Autodesk Fusion 360 part; units mm, degrees
note: some values were not read from the file. Chosen so that the rebuilt part matches the saved one: which face or edge a step refers to; how an offset face is resized; which pieces of a blend or face edit are solid. Set by a fixed rule: which sketch regions a step uses.
(part 2 of 2)
sketch "Sketch41" plane through (0, 0, 152) normal (0, 0, 1) x (-1, 0, 0)
  circle A0 centre (0, 0) radius 37.5
  circle A1 centre (-35, 35) radius 4.5178
  circle A2 centre (35, -35) radius 4.5178
  circle A3 centre (35, 35) radius 4.5178
  circle A4 centre (-35, -35) radius 4.5178
  line L0 (-250.7522, -75) -> (250.25, -75)
  line L1 (250.25, -75) -> (250.25, 75)
  line L2 (250.25, 75) -> (-250.7522, 75)
  line L3 (-250.7522, 75) -> (-250.7522, -75)
  line L4 (250.25, -75) -> (237.75, -75)
  line L5 (237.75, -75) -> (237.75, -50)
  line L6 (237.75, -50) -> (250.25, -50)
  line L7 (250.25, -50) -> (250.25, -75)
  line L8 (250.25, 75) -> (237.75, 75)
  line L9 (237.75, 75) -> (237.75, 50)
  line L10 (237.75, 50) -> (250.25, 50)
  line L11 (250.25, 50) -> (250.25, 75)
  line L12 (237.75, 50) -> (237.75, 0)
  line L13 (-250.7522, -75) -> (-238.2522, -75)
  line L14 (-238.2522, -75) -> (-238.2522, -50)
  line L15 (-238.2522, -50) -> (-250.7522, -50)
  line L16 (-250.7522, -50) -> (-250.7522, -75)
  line L17 (-250.7522, 75) -> (-238.2522, 75)
  line L18 (-238.2522, 75) -> (-238.2522, 50)
  line L19 (-238.2522, 50) -> (-250.7522, 50)
  line L20 (-250.7522, 50) -> (-250.7522, 75)
  line L21 (-238.2522, 50) -> (-238.2522, 0)
  dimension "d300" = 12.5
  dimension "d301" = 25
  dimension "d302" = 12.5
  dimension "d303" = 25
  dimension "d304" = 50
  dimension "d305" = 12.5
  dimension "d306" = 25
  dimension "d307" = 12.5
  dimension "d308" = 25
  dimension "d309" = 50
  constraint horizontal L4
  constraint vertical L5
  constraint horizontal L6
  constraint vertical L7
  constraint coincident L0.end L1.start
  constraint horizontal L8
  constraint vertical L9
  constraint horizontal L10
  constraint vertical L11
  constraint coincident L1.end L2.start
  constraint perpendicular L10 L12
  constraint horizontal L13
  constraint vertical L14
  constraint horizontal L15
  constraint vertical L16
  constraint coincident L0.start L3.end
  constraint horizontal L17
  constraint vertical L18
  constraint horizontal L19
  constraint vertical L20
  constraint coincident L2.end L3.start
  constraint perpendicular L19 L21
  measures "d300" distance of L0.end L4.end
  measures "d301" distance of L0.end L6.end
  measures "d302" distance of L1.end L8.end
  measures "d303" distance of L1.end L10.end
  measures "d304" distance of L9.end L12.end
  measures "d305" distance of L0.start L13.end
  measures "d306" distance of L0.start L15.end
  measures "d307" distance of L2.end L17.end
  measures "d308" distance of L2.end L19.end
  measures "d309" distance of L18.end L21.end
hole "Hole23" at (238.2522, 50, 152) at (238.2522, 0, 152) at (238.2522, -50, 152) at (-237.75, -50, 152) at (-237.75, 0, 152) at (-237.75, 50, 152) direction (0, 0, -1) diameter 9 depth 60 tip angle 180
extrude "Extrude48" cut 1 faces at (250.7522, -25, 135.3333) along direction (-1, 0, 0) blind 0.502
delete_face "DeleteFace35" 1 faces at (239.7913, -45.7714, 143.6667)
delete_face "DeleteFace36" 1 faces at (238.4765, -4.4944, 143.6667)
delete_face "DeleteFace37" 1 faces at (239.7913, 54.2286, 143.6667)
sketch "Sketch42" plane through (0, 0, 152) normal (0, 0, 1) x (-1, 0, 0)
  line L0 (-250.2502, 75) -> (-250.2502, -75)
  line L1 (-250.2502, -75) -> (250.25, -75)
  line L2 (250.25, -75) -> (250.25, 75)
  line L3 (250.25, 75) -> (-250.2502, 75)
  circle A0 centre (237.75, 0) radius 4.5
  circle A1 centre (237.75, 50) radius 4.5
  circle A2 centre (237.75, -50) radius 4.5
  circle A3 centre (0, 0) radius 37.5
  circle A4 centre (-35, 35) radius 4.5178
  circle A5 centre (35, -35) radius 4.5178
  circle A6 centre (35, 35) radius 4.5178
  circle A7 centre (-35, -35) radius 4.5178
  line L4 (-250.2502, -75) -> (-237.7502, -75)
  line L5 (-237.7502, -75) -> (-237.7502, -50)
  line L6 (-237.7502, -50) -> (-250.2502, -50)
  line L7 (-250.2502, -50) -> (-250.2502, -75)
  line L8 (-250, 75) -> (-237.5, 75)
  line L9 (-237.5, 75) -> (-237.5, 50)
  line L10 (-237.5, 50) -> (-250, 50)
  line L11 (-250, 50) -> (-250, 75)
  line L12 (-237.5, 50) -> (-237.5, 0)
  dimension "d315" = 12.5
  dimension "d316" = 25
  dimension "d317" = 12.5
  dimension "d318" = 25
  dimension "d319" = 50
  constraint horizontal L4
  constraint vertical L5
  constraint horizontal L6
  constraint vertical L7
  constraint coincident L0.end L1.start
  constraint horizontal L8
  constraint vertical L9
  constraint horizontal L10
  constraint vertical L11
  constraint perpendicular L10 L12
  measures "d315" distance of L0.end L4.end
  measures "d316" distance of L0.end L6.end
  measures "d317" distance of L8.start L8.end
  measures "d318" distance of L8.start L10.end
  measures "d319" distance of L9.end L12.end
hole "Hole24" at (237.7502, 50, 152) at (237.5, 0, 152) at (237.5, -50, 152) direction (0, 0, -1) diameter 9 depth 60 tip angle 180
delete_face "DeleteFace38" 1 faces at (239.0391, -45.7714, 143.6667)
delete_face "DeleteFace39" 1 faces at (239.0391, 4.2286, 143.6667)
sketch "Sketch43" plane through (0, 0, 152) normal (0, 0, 1) x (-1, 0, 0)
  circle A0 centre (-237.7502, -50) radius 4.5
  line L0 (-250.2502, 75) -> (-250.2502, -75)
  line L1 (-250.2502, -75) -> (250.25, -75)
  line L2 (250.25, -75) -> (250.25, 75)
  line L3 (250.25, 75) -> (-250.2502, 75)
  circle A1 centre (237.75, 0) radius 4.5
  circle A2 centre (237.75, 50) radius 4.5
  circle A3 centre (237.75, -50) radius 4.5
  circle A4 centre (0, 0) radius 37.5
  circle A5 centre (-35, 35) radius 4.5178
  circle A6 centre (35, -35) radius 4.5178
  circle A7 centre (35, 35) radius 4.5178
  circle A8 centre (-35, -35) radius 4.5178
  line L4 (-237.7502, -50) -> (-237.7502, 0)
  line L5 (-237.7502, 0) -> (-237.7502, 50)
  dimension "d323" = 50
  dimension "d324" = 50
  constraint coincident A0.centre L4.start
  constraint parallel L0 L4
  constraint vertical L5
  measures "d323" distance of A0.centre L4.end
  measures "d324" distance of L4.end L5.end
hole "Hole25" at (237.7502, 0, 152) at (237.7502, -50, 152) direction (0, 0, -1) diameter 9 depth 60 tip angle 180
extrude "Extrude49" cut 1 faces at (167.9358, -18.5297, 127) along direction (0, 0, 1) blind 5
sketch "Sketch44" plane through (0, -75, 0) normal (0, -1, 0) x (1, 0, 0)
  line L0 (-250.25, 132) -> (250.2502, 132)
  line L1 (250.2502, 132) -> (250.2502, 152)
  line L2 (250.2502, 152) -> (-250.25, 152)
  line L3 (-250.25, 152) -> (-250.25, 132)
  line L4 (0.0001, 152) -> (40.0001, 152)
  line L5 (40.0001, 152) -> (40.0001, 145)
  line L6 (40.0001, 145) -> (0.0001, 145)
  line L7 (0.0001, 145) -> (0.0001, 152)
  line L8 (40.0001, 145) -> (80.0001, 145)
  line L9 (80.0001, 145) -> (120.0001, 145)
  line L10 (120.0001, 145) -> (160.0001, 145)
  dimension "d330" = 40
  dimension "d331" = 7
  dimension "d332" = 40
  dimension "d333" = 40
  dimension "d334" = 40
  constraint horizontal L4
  constraint vertical L5
  constraint horizontal L6
  constraint vertical L7
  constraint midpoint L2 L4.start
  constraint perpendicular L5 L8
  constraint parallel L8 L9
  constraint horizontal L10
  measures "d330" distance of L4.start L4.end
  measures "d331" distance of L4.start L6.end
  measures "d332" distance of L5.end L8.end
  measures "d333" distance of L8.end L9.end
  measures "d334" distance of L9.end L10.end
sketch "Sketch45" plane through (0, 75, 0) normal (0, 1, 0) x (-1, 0, 0)
  line L0 (-250.2502, 132) -> (250.25, 132)
  line L1 (250.25, 132) -> (250.25, 152)
  line L2 (250.25, 152) -> (-250.2502, 152)
  line L3 (-250.2502, 152) -> (-250.2502, 132)
  line L4 (-0.0001, 152) -> (-40.0001, 152)
  line L5 (-40.0001, 152) -> (-40.0001, 145)
  line L6 (-40.0001, 145) -> (-0.0001, 145)
  line L7 (-0.0001, 145) -> (-0.0001, 152)
  line L8 (-40.0001, 145) -> (-80.0001, 145)
  line L9 (-80.0001, 145) -> (-120.0001, 145)
  line L10 (-120.0001, 145) -> (-160.0001, 145)
  dimension "d338" = 40
  dimension "d339" = 7
  dimension "d340" = 40
  dimension "d341" = 40
  dimension "d342" = 40
  constraint horizontal L4
  constraint vertical L5
  constraint horizontal L6
  constraint vertical L7
  constraint midpoint L2 L4.start
  constraint perpendicular L5 L8
  constraint parallel L8 L9
  constraint parallel L9 L10
  measures "d338" distance of L4.start L4.end
  measures "d339" distance of L4.start L6.end
  measures "d340" distance of L5.end L8.end
  measures "d341" distance of L8.end L9.end
  measures "d342" distance of L9.end L10.end
sketch "Sketch46" plane through (0, 0, 152) normal (0, 0, 1) x (-1, 0, 0)
  circle A0 centre (-237.7502, 0) radius 4.5
  circle A1 centre (-237.7502, 50) radius 4.5
  circle A2 centre (-237.7502, -50) radius 4.5
  line L0 (-250.2502, 75) -> (-250.2502, -75)
  line L1 (-250.2502, -75) -> (250.25, -75)
  line L2 (250.25, -75) -> (250.25, 75)
  line L3 (250.25, 75) -> (-250.2502, 75)
  circle A3 centre (237.75, 0) radius 4.5
  circle A4 centre (237.75, 50) radius 4.5
  circle A5 centre (237.75, -50) radius 4.5
  circle A6 centre (0, 0) radius 37.5
  circle A7 centre (-35, 35) radius 4.5178
  circle A8 centre (35, -35) radius 4.5178
  circle A9 centre (35, 35) radius 4.5178
  circle A10 centre (-35, -35) radius 4.5178
  line L4 (-191.7562, -13.746) -> (-196.7562, -13.746)
  line L5 (-196.7562, -13.746) -> (-224.2482, -13.746)
  line L6 (-224.2482, -13.746) -> (-224.2482, 13.746)
  line L7 (-224.2482, 13.746) -> (-196.7562, 13.746)
  line L8 (-196.7562, 13.746) -> (-196.7562, -13.746)
  dimension "d346" = 5
  dimension "d347" = 27.492
  dimension "d348" = 27.492
  constraint horizontal L4
  constraint horizontal L5
  constraint vertical L6
  constraint horizontal L7
  constraint vertical L8
  measures "d346" distance of L4.start L4.end
  measures "d347" distance of L4.end L5.end
  measures "d348" distance of L4.end L7.end
hole "Hole28" at (196.7562, 13.746, 152) at (196.7562, -13.746, 152) at (224.2482, -13.746, 152) at (224.2482, 13.746, 152) direction (0, 0, -1) diameter 5.035 depth 10 tip angle 180
thread "Thread23" "ISO Metric profile 6.0 M6x1 6H"
sketch "Sketch47" plane through (0, 0, 152) normal (0, 0, 1) x (-1, 0, 0)
  circle A0 centre (-224.2482, 13.746) radius 2.5175
  circle A1 centre (-196.7562, -13.746) radius 2.5175
  circle A2 centre (-196.7562, 13.746) radius 2.5175
  circle A3 centre (-224.2482, -13.746) radius 2.5175
  circle A4 centre (-237.7502, 0) radius 4.5
  circle A5 centre (-237.7502, 50) radius 4.5
  circle A6 centre (-237.7502, -50) radius 4.5
  line L0 (-250.2502, 75) -> (-250.2502, -75)
  line L1 (-250.2502, -75) -> (250.25, -75)
  line L2 (250.25, -75) -> (250.25, 75)
  line L3 (250.25, 75) -> (-250.2502, 75)
  circle A7 centre (237.75, 0) radius 4.5
  circle A8 centre (237.75, 50) radius 4.5
  circle A9 centre (237.75, -50) radius 4.5
  circle A10 centre (0, 0) radius 37.5
  circle A11 centre (-35, 35) radius 4.5178
  circle A12 centre (35, -35) radius 4.5178
  circle A13 centre (35, 35) radius 4.5178
  circle A14 centre (-35, -35) radius 4.5178
  circle A15 centre (0, 0) radius 35
  dimension "d352" = 70
  constraint coincident A10.centre A15.centre
  measures "d352" diameter of A15
extrude "Extrude50" add sketch "Sketch47" against normal blind 20 contours A10
sketch "Sketch48" plane through (0, 0, 152) normal (0, 0, 1) x (-1, 0, 0)
  circle A0 centre (0, 0) radius 35
  circle A1 centre (-224.2482, 13.746) radius 2.5175
  circle A2 centre (-196.7562, -13.746) radius 2.5175
  circle A3 centre (-196.7562, 13.746) radius 2.5175
  circle A4 centre (-224.2482, -13.746) radius 2.5175
  circle A5 centre (-237.7502, 0) radius 4.5
  circle A6 centre (-237.7502, 50) radius 4.5
  circle A7 centre (-237.7502, -50) radius 4.5
  line L0 (-250.2502, 75) -> (-250.2502, -75)
  line L1 (-250.2502, -75) -> (250.25, -75)
  line L2 (250.25, -75) -> (250.25, 75)
  line L3 (250.25, 75) -> (-250.2502, 75)
  circle A8 centre (237.75, 0) radius 4.5
  circle A9 centre (237.75, 50) radius 4.5
  circle A10 centre (237.75, -50) radius 4.5
  circle A11 centre (-35, 35) radius 4.5178
  circle A12 centre (35, -35) radius 4.5178
  circle A13 centre (35, 35) radius 4.5178
  circle A14 centre (-35, -35) radius 4.5178
  circle A15 centre (0, 0) radius 40
  dimension "d355" = 80
  constraint coincident A0.centre A15.centre
  measures "d355" diameter of A15
extrude "Extrude51" cut sketch "Sketch48" against normal blind 35 contours A15
extrude "Extrude52" add 1 faces at (-168.7478, 28.3333, 152) along direction (0, 0, 1) blind 5
delete_face "DeleteFace40" 2 faces at (-34.7748, 30.4879, 153.6667) (-36.2773, 34.7238, 147)
delete_face "DeleteFace41" 3 faces at (-34.7748, -39.5121, 155.3333) (-34.5502, -39.4953, 148.6667) (-36.2773, -35.2762, 147)
delete_face "DeleteFace42" 2 faces at (35.2252, -39.5121, 153.6667) (33.7227, -35.2762, 147)
delete_face "DeleteFace43" 2 faces at (35.2252, 30.4879, 153.6667) (33.7227, 34.7238, 147)
sketch "Sketch49" plane through (0, 0, 157) normal (0, 0, 1) x (-1, 0, 0)
  circle A0 centre (0, 0) radius 40
  circle A1 centre (-224.2482, 13.746) radius 2.5175
  circle A2 centre (-196.7562, -13.746) radius 2.5175
  circle A3 centre (-196.7562, 13.746) radius 2.5175
  circle A4 centre (-224.2482, -13.746) radius 2.5175
  circle A5 centre (-237.7502, 0) radius 4.5
  circle A6 centre (-237.7502, 50) radius 4.5
  circle A7 centre (-237.7502, -50) radius 4.5
  line L0 (-250.2502, 75) -> (-250.2502, -75)
  line L1 (-250.2502, -75) -> (250.25, -75)
  line L2 (250.25, -75) -> (250.25, 75)
  line L3 (250.25, 75) -> (-250.2502, 75)
  circle A8 centre (237.75, 0) radius 4.5
  circle A9 centre (237.75, 50) radius 4.5
  circle A10 centre (237.75, -50) radius 4.5
  line L4 (0, 0) -> (-35, 0)
  line L5 (-35, 0) -> (-35, -35)
  line L6 (-35, -35) -> (0, -35)
  line L7 (0, -35) -> (0, 0)
  line L8 (-35, -35) -> (35, -35)
  line L9 (35, -35) -> (35, 35)
  line L10 (35, 35) -> (-35, 35)
  line L11 (-35, 35) -> (-35, -35)
  dimension "d360" = 35
  dimension "d361" = 35
  dimension "d362" = 70
  dimension "d363" = 70
  constraint horizontal L4
  constraint vertical L5
  constraint horizontal L6
  constraint vertical L7
  constraint coincident A0.centre L4.start
  constraint horizontal L8
  constraint vertical L9
  constraint horizontal L10
  constraint vertical L11
  measures "d360" distance of A0.centre L4.end
  measures "d361" distance of A0.centre L6.end
  measures "d362" distance of L5.end L8.end
  measures "d363" distance of L5.end L10.end
hole "Hole29" at (-35, 35, 157) at (-35, -35, 157) at (35, -35, 157) at (35, 35, 157) direction (0, 0, -1) diameter 10.274 depth 80 tip angle 180
thread "Thread24" "ISO Metric profile 12.0 M12x1 6H" major diameter 12.152 minor diameter 11.035 pitch 1 angle 60 resizes the face on face at (-34.4885, 29.8885, 140.3333) on face at (-34.4885, -40.1115, 140.3333) on face at (35.5115, -40.1115, 140.3333) on face at (35.5115, 29.8885, 140.3333)
extrude "Extrude53" add 4 faces at (223.4484, 13.6889, 142) (195.9564, 13.6889, 142) (224.9683, -15.2412, 142) (197.4763, -15.2412, 142) along direction (0, 0, 1) blind 5
sketch "Sketch50" plane through (0, 0, 157) normal (0, 0, 1) x (-1, 0, 0)
  circle A0 centre (-35, 35) radius 5.5175
  circle A1 centre (35, -35) radius 5.5175
  circle A2 centre (35, 35) radius 5.5175
  circle A3 centre (-35, -35) radius 5.5175
  circle A4 centre (0, 0) radius 40
  circle A5 centre (-224.2482, 13.746) radius 2.5175
  circle A6 centre (-196.7562, -13.746) radius 2.5175
  circle A7 centre (-196.7562, 13.746) radius 2.5175
  circle A8 centre (-224.2482, -13.746) radius 2.5175
  circle A9 centre (-237.7502, 0) radius 4.5
  circle A10 centre (-237.7502, 50) radius 4.5
  circle A11 centre (-237.7502, -50) radius 4.5
  line L0 (-250.2502, 75) -> (-250.2502, -75)
  line L1 (-250.2502, -75) -> (250.25, -75)
  line L2 (250.25, -75) -> (250.25, 75)
  line L3 (250.25, 75) -> (-250.2502, 75)
  circle A12 centre (237.75, 0) radius 4.5
  circle A13 centre (237.75, 50) radius 4.5
  circle A14 centre (237.75, -50) radius 4.5
  circle A15 centre (0, 0) radius 35
  dimension "d369" = 70
  constraint coincident A4.centre A15.centre
  measures "d369" diameter of A15
extrude "Extrude54" add sketch "Sketch50" against normal blind 25 contours A4
delete_face "DeleteFace44" 1 faces at (222.2042, 12.2764, 150.3333)
delete_face "DeleteFace45" 1 faces at (194.7122, 12.2764, 150.3333)
delete_face "DeleteFace46" 2 faces at (195.8952, -16.1117, 153.6667) (197.4763, -15.2412, 147)
delete_face "DeleteFace47" 1 faces at (223.3872, -16.1117, 153.6667)
sketch "Sketch51" plane through (0, 0, 157) normal (0, 0, 1) x (-1, 0, 0)
  circle A0 centre (0, 0) radius 35
  circle A1 centre (-35, 35) radius 5.5175
  circle A2 centre (35, -35) radius 5.5175
  circle A3 centre (35, 35) radius 5.5175
  circle A4 centre (-35, -35) radius 5.5175
  circle A5 centre (-237.7502, 0) radius 4.5
  circle A6 centre (-237.7502, 50) radius 4.5
  circle A7 centre (-237.7502, -50) radius 4.5
  line L0 (-250.2502, 75) -> (-250.2502, -75)
  line L1 (-250.2502, -75) -> (250.25, -75)
  line L2 (250.25, -75) -> (250.25, 75)
  line L3 (250.25, 75) -> (-250.2502, 75)
  circle A8 centre (237.75, 0) radius 4.5
  circle A9 centre (237.75, 50) radius 4.5
  circle A10 centre (237.75, -50) radius 4.5
  line L4 (-250, 0) -> (-220, 0)
  line L5 (-219.5619, 0) -> (-204.5619, 0)
  line L6 (-204.5619, 0) -> (-204.5619, -15)
  line L7 (-204.5619, -15) -> (-219.5619, -15)
  line L8 (-219.5619, -15) -> (-219.5619, 0)
  line L9 (-219.5619, -15) -> (-189.5619, -15)
  line L10 (-189.5619, -15) -> (-189.5619, 15)
  line L11 (-189.5619, 15) -> (-219.5619, 15)
  line L12 (-219.5619, 15) -> (-219.5619, -15)
  dimension "d372" = 30
  dimension "d373" = 15
  dimension "d374" = 15
  dimension "d375" = 30
  dimension "d376" = 30
  constraint perpendicular L0 L4
  constraint horizontal L5
  constraint vertical L6
  constraint horizontal L7
  constraint vertical L8
  constraint horizontal L9
  constraint vertical L10
  constraint horizontal L11
  constraint vertical L12
  measures "d372" distance of L4.start L4.end
  measures "d373" distance of L5.start L5.end
  measures "d374" distance of L5.start L7.end
  measures "d375" distance of L7.end L9.end
  measures "d376" distance of L7.end L11.end
sketch "Sketch52" plane through (0, 0, 157) normal (0, 0, 1) x (-1, 0, 0)
  circle A0 centre (0, 0) radius 35
  circle A1 centre (-35, 35) radius 5.5175
  circle A2 centre (35, -35) radius 5.5175
  circle A3 centre (35, 35) radius 5.5175
  circle A4 centre (-35, -35) radius 5.5175
  circle A5 centre (-237.7502, 0) radius 4.5
  circle A6 centre (-237.7502, 50) radius 4.5
  circle A7 centre (-237.7502, -50) radius 4.5
  line L0 (-250.2502, 75) -> (-250.2502, -75)
  line L1 (-250.2502, -75) -> (250.25, -75)
  line L2 (250.25, -75) -> (250.25, 75)
  line L3 (250.25, 75) -> (-250.2502, 75)
  circle A8 centre (237.75, 0) radius 4.5
  circle A9 centre (237.75, 50) radius 4.5
  circle A10 centre (237.75, -50) radius 4.5
  line L4 (-250.2502, 0) -> (-220.2502, 0)
  line L5 (-220.2502, 0) -> (-205.2502, 0)
  line L6 (-205.2502, 0) -> (-205.2502, 15)
  line L7 (-205.2502, 15) -> (-220.2502, 15)
  line L8 (-220.2502, 15) -> (-220.2502, 0)
  line L9 (-220.2502, 15) -> (-190.2502, 15)
  line L10 (-190.2502, 15) -> (-190.2502, -15)
  line L11 (-190.2502, -15) -> (-220.2502, -15)
  line L12 (-220.2502, -15) -> (-220.2502, 15)
  dimension "d380" = 30
  dimension "d381" = 15
  dimension "d382" = 15
  dimension "d383" = 30
  dimension "d384" = 30
  constraint midpoint L0 L4.start
  constraint perpendicular L0 L4
  constraint horizontal L5
  constraint vertical L6
  constraint horizontal L7
  constraint vertical L8
  constraint horizontal L9
  constraint vertical L10
  constraint horizontal L11
  constraint vertical L12
  measures "d380" distance of L4.start L4.end
  measures "d381" distance of L4.end L5.end
  measures "d382" distance of L4.end L7.end
  measures "d383" distance of L7.end L9.end
  measures "d384" distance of L7.end L11.end
sketch "Sketch53" plane through (0, 0, 157) normal (0, 0, 1) x (-1, 0, 0)
  circle A0 centre (0, 0) radius 35
  circle A1 centre (-35, 35) radius 5.5175
  circle A2 centre (35, -35) radius 5.5175
  circle A3 centre (35, 35) radius 5.5175
  circle A4 centre (-35, -35) radius 5.5175
  circle A5 centre (-237.7502, 0) radius 4.5
  circle A6 centre (-237.7502, 50) radius 4.5
  circle A7 centre (-237.7502, -50) radius 4.5
  line L0 (-250.2502, 75) -> (-250.2502, -75)
  line L1 (-250.2502, -75) -> (250.25, -75)
  line L2 (250.25, -75) -> (250.25, 75)
  line L3 (250.25, 75) -> (-250.2502, 75)
  circle A8 centre (237.75, 0) radius 4.5
  circle A9 centre (237.75, 50) radius 4.5
  circle A10 centre (237.75, -50) radius 4.5
  line L4 (-190.2502, -15) -> (-194.2502, -15)
  line L5 (-194.2502, -15) -> (-224.2502, -15)
  line L6 (-224.2502, -15) -> (-224.2502, 15)
  line L7 (-224.2502, 15) -> (-194.2502, 15)
  line L8 (-194.2502, 15) -> (-194.2502, -15)
  dimension "d388" = 4
  dimension "d389" = 30
  dimension "d390" = 30
  constraint horizontal L4
  constraint horizontal L5
  constraint vertical L6
  constraint horizontal L7
  constraint vertical L8
  measures "d388" distance of L4.start L4.end
  measures "d389" distance of L4.end L5.end
  measures "d390" distance of L4.end L7.end
sketch "Sketch54" plane through (0, 0, 157) normal (0, 0, 1) x (-1, 0, 0)
  circle A0 centre (0, 0) radius 35
  circle A1 centre (-35, 35) radius 5.5175
  circle A2 centre (35, -35) radius 5.5175
  circle A3 centre (35, 35) radius 5.5175
  circle A4 centre (-35, -35) radius 5.5175
  circle A5 centre (-237.7502, 0) radius 4.5
  circle A6 centre (-237.7502, 50) radius 4.5
  circle A7 centre (-237.7502, -50) radius 4.5
  line L0 (-250.2502, 75) -> (-250.2502, -75)
  line L1 (-250.2502, -75) -> (250.25, -75)
  line L2 (250.25, -75) -> (250.25, 75)
  line L3 (250.25, 75) -> (-250.2502, 75)
  circle A8 centre (237.75, 0) radius 4.5
  circle A9 centre (237.75, 50) radius 4.5
  circle A10 centre (237.75, -50) radius 4.5
  line L4 (-224.2502, 15) -> (-222.9942, 15)
  line L5 (-222.9942, 15) -> (-192.9942, 15)
  line L6 (-192.9942, 15) -> (-192.9942, -15)
  line L7 (-192.9942, -15) -> (-222.9942, -15)
  line L8 (-222.9942, -15) -> (-222.9942, 15)
  dimension "d394" = 1.256
  dimension "d395" = 30
  dimension "d396" = 30
  constraint horizontal L4
  constraint horizontal L5
  constraint vertical L6
  constraint horizontal L7
  constraint vertical L8
  measures "d394" distance of L4.start L4.end
  measures "d395" distance of L4.end L5.end
  measures "d396" distance of L4.end L7.end
hole "Hole33" at (192.9942, -15, 157) at (222.9942, -15, 157) at (222.9942, 15, 157) at (192.9942, 15, 157) direction (0, 0, -1) diameter 5.035 depth 10 tip angle 180
thread "Thread28" "ISO Metric profile 6.0 M6x1 6H"
delete_face "DeleteFace48" 2 faces at (222.1332, -17.3657, 153.6667) (223.7143, -16.4952, 147)
delete_face "DeleteFace49" 1 faces at (225.0383, 16.4696, 153.6667)
delete_face "DeleteFace50" 1 faces at (195.0383, 16.4696, 153.6667)
delete_face "DeleteFace51" 1 faces at (192.1332, -17.3657, 153.6667)
sketch "Sketch55" plane through (0, 0, 157) normal (0, 0, 1) x (-1, 0, 0)
  circle A0 centre (0, 0) radius 35
  circle A1 centre (-35, 35) radius 5.5175
  circle A2 centre (35, -35) radius 5.5175
  circle A3 centre (35, 35) radius 5.5175
  circle A4 centre (-35, -35) radius 5.5175
  circle A5 centre (-237.7502, 0) radius 4.5
  circle A6 centre (-237.7502, 50) radius 4.5
  circle A7 centre (-237.7502, -50) radius 4.5
  line L0 (-250.2502, 75) -> (-250.2502, -75)
  line L1 (-250.2502, -75) -> (250.25, -75)
  line L2 (250.25, -75) -> (250.25, 75)
  line L3 (250.25, 75) -> (-250.2502, 75)
  circle A8 centre (237.75, 0) radius 4.5
  circle A9 centre (237.75, 50) radius 4.5
  circle A10 centre (237.75, -50) radius 4.5
  line L4 (-250.2502, 0) -> (-220.2502, 0)
  line L5 (-220.2502, 0) -> (-205.2502, 0)
  line L6 (-205.2502, 0) -> (-205.2502, 15)
  line L7 (-205.2502, 15) -> (-220.2502, 15)
  line L8 (-220.2502, 15) -> (-220.2502, 0)
  line L9 (-220.2502, 15) -> (-190.2502, 15)
  line L10 (-190.2502, 15) -> (-190.2502, -15)
  line L11 (-190.2502, -15) -> (-220.2502, -15)
  line L12 (-220.2502, -15) -> (-220.2502, 15)
  dimension "d400" = 30
  dimension "d401" = 15
  dimension "d402" = 15
  dimension "d403" = 30
  dimension "d404" = 30
  constraint midpoint L0 L4.start
  constraint perpendicular L0 L4
  constraint horizontal L5
  constraint vertical L6
  constraint horizontal L7
  constraint vertical L8
  constraint horizontal L9
  constraint vertical L10
  constraint horizontal L11
  constraint vertical L12
  measures "d400" distance of L4.start L4.end
  measures "d401" distance of L4.end L5.end
  measures "d402" distance of L4.end L7.end
  measures "d403" distance of L7.end L9.end
  measures "d404" distance of L7.end L11.end
hole "Hole34" at (220.2502, -15, 157) at (220.2502, 15, 157) at (190.2502, 15, 157) at (190.2502, -15, 157) direction (0, 0, -1) diameter 5.035 depth 10 tip angle 180
thread "Thread29" "ISO Metric profile 6.0 M6x1 6H"
sketch "Sketch56" plane through (0, 0, 157) normal (0, 0, 1) x (-1, 0, 0)
  circle A0 centre (-190.2502, -15) radius 2.5175
  circle A1 centre (-220.2502, 15) radius 2.5175
  circle A2 centre (-220.2502, -15) radius 2.5175
  circle A3 centre (-190.2502, 15) radius 2.5175
  circle A4 centre (0, 0) radius 35
  circle A5 centre (-35, 35) radius 5.5175
  circle A6 centre (35, -35) radius 5.5175
  circle A7 centre (35, 35) radius 5.5175
  circle A8 centre (-35, -35) radius 5.5175
  circle A9 centre (-237.7502, 0) radius 4.5
  circle A10 centre (-237.7502, 50) radius 4.5
  circle A11 centre (-237.7502, -50) radius 4.5
  line L0 (-250.2502, 75) -> (-250.2502, -75)
  line L1 (-250.2502, -75) -> (250.25, -75)
  line L2 (250.25, -75) -> (250.25, 75)
  line L3 (250.25, 75) -> (-250.2502, 75)
  circle A12 centre (237.75, 0) radius 4.5
  circle A13 centre (237.75, 50) radius 4.5
  circle A14 centre (237.75, -50) radius 4.5
  line L4 (-220.2502, -15) -> (-205.2502, -15)
  line L5 (-205.2502, -15) -> (-205.2502, -13.9091)
  line L6 (-205.2502, -13.9091) -> (-205.2502, 16.0909)
  dimension "d408" = 15
  dimension "d409" = 30
  constraint coincident A2.centre L4.start
  constraint horizontal L4
  constraint perpendicular L4 L5
  constraint perpendicular L4 L6
  measures "d408" distance of A2.centre L4.end
  measures "d409" distance of L5.end L6.end
hole "Hole35" at (205.2502, 15, 157) at (205.2502, -16.0909, 157) direction (0, 0, -1) diameter 5.035 depth 10 tip angle 180
thread "Thread30" "ISO Metric profile 6.0 M6x1 6H"
delete_face "DeleteFace52" 2 faces at (188.1355, 13.6341, 153.6667) (189.4504, 15.4306, 147)
delete_face "DeleteFace53" 2 faces at (189.3892, -17.3657, 153.6667) (190.9703, -16.4952, 147)
delete_face "DeleteFace54" 2 faces at (204.3892, -18.4566, 153.6667) (205.9703, -17.5862, 147)
sketch "Sketch57" plane through (0, 0, 157) normal (0, 0, 1) x (-1, 0, 0)
  circle A0 centre (-205.2502, -15) radius 2.5175
  circle A1 centre (-220.2502, 15) radius 2.5175
  circle A2 centre (-220.2502, -15) radius 2.5175
  circle A3 centre (0, 0) radius 35
  circle A4 centre (-35, 35) radius 5.5175
  circle A5 centre (35, -35) radius 5.5175
  circle A6 centre (35, 35) radius 5.5175
  circle A7 centre (-35, -35) radius 5.5175
  circle A8 centre (-237.7502, 0) radius 4.5
  circle A9 centre (-237.7502, 50) radius 4.5
  circle A10 centre (-237.7502, -50) radius 4.5
  line L0 (-250.2502, 75) -> (-250.2502, -75)
  line L1 (-250.2502, -75) -> (250.25, -75)
  line L2 (250.25, -75) -> (250.25, 75)
  line L3 (250.25, 75) -> (-250.2502, 75)
  circle A11 centre (237.75, 0) radius 4.5
  circle A12 centre (237.75, 50) radius 4.5
  circle A13 centre (237.75, -50) radius 4.5
  line L4 (-220.2502, 15) -> (-205.2502, 15)
  dimension "d413" = 15
  constraint coincident A1.centre L4.start
  constraint horizontal L4
  measures "d413" distance of A1.centre L4.end
hole "Hole36" at (205.2502, -15, 157) direction (0, 0, -1) diameter 5.035 depth 10 tip angle 180
thread "Thread31" "ISO Metric profile 6.0 M6x1 6H"
sketch "Sketch58" plane through (0, -75, 0) normal (0, -1, 0) x (1, 0, 0)
  line L0 (-250.25, 132) -> (250.2502, 132)
  line L1 (250.2502, 132) -> (250.2502, 157)
  line L2 (250.2502, 157) -> (-250.25, 157)
  line L3 (-250.25, 157) -> (-250.25, 132)
  line L4 (40.0001, 145) -> (40.0001, 150)
  line L5 (40.0001, 150) -> (80.0001, 150)
  line L6 (80.0001, 150) -> (120.0001, 150)
  line L7 (120.0001, 150) -> (160.0001, 150)
  dimension "d417" = 5
  dimension "d418" = 40
  dimension "d419" = 40
  dimension "d420" = 40
  constraint perpendicular L2 L4
  constraint perpendicular L4 L5
  constraint horizontal L6
  constraint parallel L6 L7
  measures "d417" distance of L4.start L4.end
  measures "d418" distance of L4.end L5.end
  measures "d419" distance of L5.end L6.end
  measures "d420" distance of L6.end L7.end
sketch "Sketch59" plane through (0, 75, 0) normal (0, 1, 0) x (-1, 0, 0)
  line L0 (-250.2502, 132) -> (250.25, 132)
  line L1 (250.25, 132) -> (250.25, 157)
  line L2 (250.25, 157) -> (-250.2502, 157)
  line L3 (-250.2502, 157) -> (-250.2502, 132)
  line L4 (-40.0001, 145) -> (-40.0001, 150)
  line L5 (-40.0001, 150) -> (-80.0001, 150)
  line L6 (-80.0001, 150) -> (-120.0001, 150)
  line L7 (-120.0001, 150) -> (-160.0001, 150)
  dimension "d424" = 5
  dimension "d425" = 40
  dimension "d426" = 40
  dimension "d427" = 40
  constraint vertical L4
  constraint perpendicular L4 L5
  constraint parallel L5 L6
  constraint parallel L6 L7
  measures "d424" distance of L4.start L4.end
  measures "d425" distance of L4.end L5.end
  measures "d426" distance of L5.end L6.end
  measures "d427" distance of L6.end L7.end
sketch "Sketch60" plane through (0, -75, 0) normal (0, -1, 0) x (1, 0, 0)
  line L0 (-250.25, 132) -> (250.2502, 132)
  line L1 (250.2502, 132) -> (250.2502, 157)
  line L2 (250.2502, 157) -> (-250.25, 157)
  line L3 (-250.25, 157) -> (-250.25, 132)
  line L4 (40.0001, 150) -> (40.0001, 147)
  line L5 (40.0001, 147) -> (80.0001, 147)
  line L6 (80.0001, 147) -> (120, 147)
  line L7 (120, 147) -> (160, 147)
  dimension "d431" = 3
  dimension "d432" = 40
  constraint vertical L4
  constraint perpendicular L4 L5
  constraint parallel L5 L6
  constraint parallel L6 L7
  measures "d431" distance of L4.start L4.end
  measures "d432" distance of L4.end L5.end
hole "Hole39" at (40.0001, -75, 147) at (80.0001, -75, 147) at (120, -75, 147) at (160, -75, 147) direction (0, 1, 0) diameter 5.035 depth 10 tip angle 180
thread "Thread34" "ISO Metric profile 6.0 M6x1 6H"
sketch "Sketch61" plane through (0, 75, 0) normal (0, 1, 0) x (-1, 0, 0)
  line L0 (-250.2502, 132) -> (250.25, 132)
  line L1 (250.25, 132) -> (250.25, 157)
  line L2 (250.25, 157) -> (-250.2502, 157)
  line L3 (-250.2502, 157) -> (-250.2502, 132)
  line L4 (-40.0001, 150) -> (-40.0001, 147)
  line L5 (-40.0001, 147) -> (-80.0001, 147)
  line L6 (-80.0001, 147) -> (-120.0001, 147)
  line L7 (-120.0001, 147) -> (-160.0001, 147)
  dimension "d436" = 3
  dimension "d437" = 40
  dimension "d438" = 40
  dimension "d439" = 40
  constraint vertical L4
  constraint perpendicular L4 L5
  constraint parallel L5 L6
  constraint parallel L6 L7
  measures "d436" distance of L4.start L4.end
  measures "d437" distance of L4.end L5.end
  measures "d438" distance of L5.end L6.end
  measures "d439" distance of L6.end L7.end
hole "Hole40" at (40.0001, 75, 147) at (80.0001, 75, 147) at (120.0001, 75, 147) at (160.0001, 75, 147) direction (0, -1, 0) diameter 5.035 depth 10 tip angle 180
thread "Thread35" "ISO Metric profile 6.0 M6x1 6H"
delete_face "DeleteFace55" 1 faces at (218.1355, 13.6341, 153.6667)
delete_face "DeleteFace56" 1 faces at (219.3892, -17.3657, 153.6667)
sketch "Sketch62" plane through (0, 0, 157) normal (0, 0, 1) x (-1, 0, 0)
  circle A0 centre (-205.2502, 15) radius 2.5175
  circle A1 centre (-205.2502, -15) radius 2.5175
  circle A2 centre (0, 0) radius 35
  circle A3 centre (-35, 35) radius 5.5175
  circle A4 centre (35, -35) radius 5.5175
  circle A5 centre (35, 35) radius 5.5175
  circle A6 centre (-35, -35) radius 5.5175
  circle A7 centre (-237.7502, 0) radius 4.5
  circle A8 centre (-237.7502, 50) radius 4.5
  circle A9 centre (-237.7502, -50) radius 4.5
  line L0 (-250.2502, 75) -> (-250.2502, -75)
  line L1 (-250.2502, -75) -> (250.25, -75)
  line L2 (250.25, -75) -> (250.25, 75)
  line L3 (250.25, 75) -> (-250.2502, 75)
  circle A10 centre (237.75, 0) radius 4.5
  circle A11 centre (237.75, 50) radius 4.5
  circle A12 centre (237.75, -50) radius 4.5
  line L4 (-250.2502, 75) -> (-195.2502, 75)
  line L5 (-195.2502, 75) -> (-195.2502, 55)
  line L6 (-195.2502, 55) -> (-250.2502, 55)
  line L7 (-250.2502, 55) -> (-250.2502, 75)
  line L8 (-250.2502, -75) -> (-195.2502, -75)
  line L9 (-195.2502, -75) -> (-195.2502, -55)
  line L10 (-195.2502, -55) -> (-250.2502, -55)
  line L11 (-250.2502, -55) -> (-250.2502, -75)
  dimension "d443" = 55
  dimension "d444" = 20
  dimension "d445" = 55
  dimension "d446" = 20
  constraint horizontal L4
  constraint vertical L5
  constraint horizontal L6
  constraint vertical L7
  constraint coincident L0.start L3.end
  constraint horizontal L8
  constraint vertical L9
  constraint horizontal L10
  constraint vertical L11
  constraint coincident L0.end L1.start
  measures "d443" distance of L0.start L4.end
  measures "d444" distance of L0.start L6.end
  measures "d445" distance of L0.end L8.end
  measures "d446" distance of L0.end L10.end
hole "Hole41" at (195.2502, 55, 157) at (195.2502, -55, 157) direction (0, 0, -1) diameter 6.78 depth 20 tip angle 180
thread "Thread36" "ISO Metric profile 8.0 M8x1 6H" major diameter 8.147 minor diameter 7.035 pitch 1 angle 60 resizes the face on face at (194.0908, 58.1856, 150.3333) on face at (194.0908, -51.8144, 150.3333)
delete_face "DeleteFace57" 1 faces at (203.2062, 13.5304, 150.3333)
delete_face "DeleteFace58" 1 faces at (204.3892, -17.3657, 153.6667)
equation "d3 = ( 215 * 2 ) * 1 mm"
equation "d137 = ( 27.492 / 2 ) * 1 mm"
equation "d146 = ( 57 / 2 ) * 1 mm"
equation "d169 = ( 1.746 * 2 ) * 1 mm"
equation "d258 = ( 490.502 / 2 ) * 1 mm"
equation "d286 = ( 57 / 2 ) * 1 mm"
